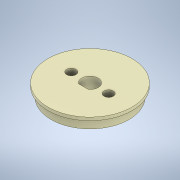
# Autodesk Inventor part: InputShaft1
Saved by Autodesk Inventor 2022 (Build 260153000, 153)
## iProperties
Created: 2022-08-30
Part Number: InputShaft1
Material: Ogólny
Document SubType Name: Modeling
Designer: MicnedSQ
Density: 1 g/cm^3
Appearance: Gładki — popielaty
Author: MicnedSQ
## iProperties of the stored document _Drukowanie 3D.ipt
Created: 2022-08-31
Part Number: _Drukowanie 3D
Material: Ogólny
Document SubType Name: Modeling
Designer: MicnedSQ
Density: 1 g/cm^3
Appearance: Domyślna
Author: MicnedSQ
Autodesk Inventor part; units mm, degrees
ref_plane "YZ Plane" through (0, 0, 0) normal (1, 0, 0) x (0, 1, 0)
ref_plane "XZ Plane" through (0, 0, 0) normal (0, 1, 0) x (-1, 0, 0)
ref_plane "XY Plane" through (0, 0, 0) normal (0, 0, 1) x (1, 0, 0)
sketch "Szkic1" plane through (0, 0, 0) normal (0, 1, 0) x (-1, 0, 0)
  circle A0 centre (0, 0) radius 12.5
  dimension "d0" = 25
  constraints: 1 centre point, 1 coincident
  measures "d0" diameter of A0
extrude "Wyciągnięcie proste1" add sketch "Szkic1" along normal blind 3
sketch "Szkic6" plane through (0, 3, 0) normal (0, 1, 0) x (1, 0, 0)
  circle A0 centre (0, 0) radius 13.5
  dimension "d13" = 27
  constraints: 1 centre point, 1 coincident
  measures "d13" diameter of A0
extrude "Wyciągnięcie proste5" add sketch "Szkic6" along normal blind 1
sketch "Szkic7" plane through (0, 4, 0) normal (0, 1, 0) x (1, 0, 0)
  point P0 (0, 0)
  point P1 (-6, 0)
  dimension "d16" = 6
  measures "d16" distance of point (-6, 0) point (0, 0)
hole "Otwór1" at (-6, 4, 0) direction (0, -1, 0) diameter 3 depth 3
pattern_circular "Szyk kołowy1" count 2 over 360 about axis through (0, 3, 0) along (0, 1, 0) of "Otwór1"
sketch "Szkic8" plane through (0, 0, 0) normal (0, -1, 0) x (1, 0, 0)
  arc A0 (-1.59, 2.12) -> (1.59, 2.12) centre (0, 0) ccw
  line L0 (1.59, 2.12) -> (-1.59, 2.12)
  dimension "d27" = 5.3
  constraints: 2 end point, 2 point on circle, 1 centre point, 1 coincident, 1 horizontal
  measures "d27" diameter of A0
extrude "Wyciągnięcie proste6" cut sketch "Szkic8" against normal through all
